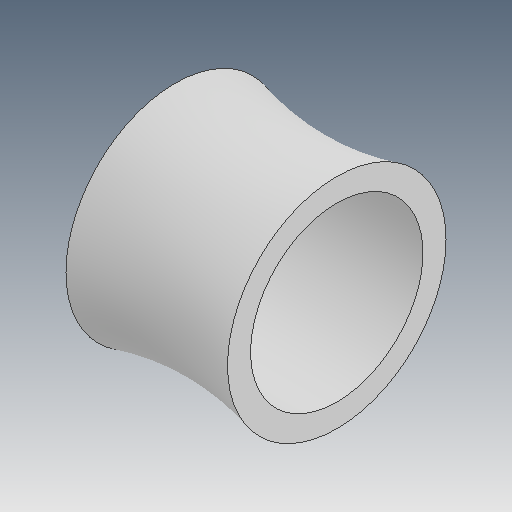
# Autodesk Inventor part: pulley_bearing_cover
Saved by Autodesk Inventor 2025.2 (Build 292293000, 293)
## iProperties
Created: 2025-02-16
Part Number: pulley_bearing_cover
Material: Generic
Document SubType Name: Modeling
Designer: email
Density: 1 g/cm^3
Appearance: Default
Author: email
Autodesk Inventor part; units mm, degrees
ref_plane "YZ Plane" through (0, 0, 0) normal (1, 0, 0) x (0, 1, 0)
ref_plane "XZ Plane" through (0, 0, 0) normal (0, 1, 0) x (-1, 0, 0)
ref_plane "XY Plane" through (0, 0, 0) normal (0, 0, 1) x (1, 0, 0)
sketch "Sketch2" plane through (0, 0, 0) normal (0, 0, 1) x (1, 0, 0)
  line L0 (-14.684, 0) -> (13.99, 0) construction
  line L1 (-10.5, 11.2) -> (10.5, 11.2)
  line L2 (10.5, 11.2) -> (10.5, 14.2)
  line L3 (-10.5, 11.2) -> (-10.5, 14.2)
  arc A0 (-10.5, 14.2) -> (10.5, 14.2) centre (0, 52.7973) ccw
  point P0 (0, 0)
  point P1 (0, 11.2)
  dimension "d0" = 22.4
  dimension "d1" = 21
  dimension "d2" = 3
  dimension "d3" = 40
  constraints: 8 end point, 2 horizontal, 2 point on circle, 1 centre point, 1 horizontal alignment, 1 midpoint, 1 perpendicular, 1 point on line, 1 vertical, 1 vertical alignment
  measures "d0" diameter of L1 L0
  measures "d1" distance between parallel lines of L2 L3
  measures "d2" distance of L1.start L3.end
  measures "d3" radius of A0
revolve "Revolution1" add sketch "Sketch2" angle 360 about axis through (-14.684, 0, 0) along (1, 0, 0)
body "Solid1"
